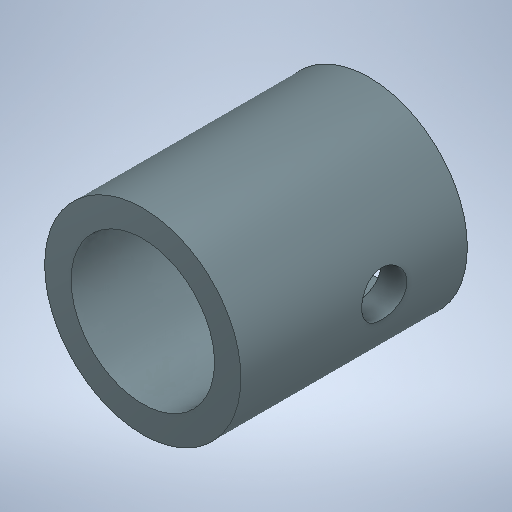
# Autodesk Inventor part: 2032
Saved by Autodesk Inventor 2025.1 (Build 291241000, 241)
## iProperties
Created: 2024-06-11
Part Number: 2032
Material: Blei
Document SubType Name: Modeling
Designer: ffogue
Density: 11.34 g/cm^3
Appearance: Blei
Author: ffogue
Autodesk Inventor part; units mm, degrees
ref_plane "XZ Plane" through (0, 0, 0) normal (0, 1, 0) x (-1, 0, 0)
ref_plane "XY Plane" through (0, 0, 0) normal (0, 0, 1) x (1, 0, 0)
sketch "Skizze1" plane through (0, 0, 0) normal (0, 1, 0) x (-1, 0, 0)
  circle A0 centre (0, 0) radius 6.5
  circle A1 centre (0, 0) radius 4.75
  dimension "d0" = 13
  dimension "d1" = 9.5
  constraints: 2 centre point, 2 coincident
  measures "d0" diameter of A0
  measures "d1" diameter of A1
extrude "Extrusion1" add sketch "Skizze1" along normal blind 15
ref_plane "Arbeitsebene1" through (6.5, 0, 0) normal (1, 0, 0) x (0, 1, 0)
sketch "Skizze2" plane through (6.5, 0, 0) normal (1, 0, 0) x (0, 1, 0)
  line L0 (0, -6.5) -> (0, 6.5) projected
  point P0 (0, 0)
  point P1 (9.5, 0)
  dimension "d5" = 9.5
  constraints: 1 horizontal alignment
  measures "d5" distance from line of L0 point (9.5, 0)
hole "Bohrung1" at (6.5, 9.5, 0) direction (-1, 0, 0) diameter 3 end through all
